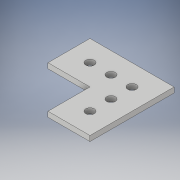
# Autodesk Inventor part: 8020 connector
Saved by Autodesk Inventor 2018 (Build 220112000, 112)
## iProperties
Created: 2019-01-26
Part Number: 8020 connector
Material: Generic
Document SubType Name: Modeling
Designer: s-2513225
Density: 1 g/cm^3
Appearance: Default
Author: s-2513225
Autodesk Inventor part; units mm, degrees
ref_plane "YZ Plane" through (0, 0, 0) normal (1, 0, 0) x (0, 1, 0)
ref_plane "XZ Plane" through (0, 0, 0) normal (0, 1, 0) x (-1, 0, 0)
ref_plane "XY Plane" through (0, 0, 0) normal (0, 0, 1) x (1, 0, 0)
sketch "Sketch1" plane through (0, 0, 0) normal (0, 1, 0) x (-1, 0, 0)
  line L0 (0, 0) -> (25.4, 0)
  line L1 (25.4, 0) -> (25.4, -25.4)
  line L2 (25.4, -50.8) -> (0, -50.8)
  line L3 (0, -50.8) -> (0, 0)
  line L4 (25.4, -50.8) -> (50.8, -50.8)
  line L5 (50.8, -50.8) -> (50.8, -25.4)
  line L6 (50.8, -25.4) -> (25.4, -25.4)
  line L7 (12.7, 0) -> (12.7, -12.7) construction
  line L8 (12.7, -12.7) -> (12.7, -25.4) construction
  line L9 (12.7, -25.4) -> (12.7, -38.1) construction
  line L10 (12.7, -38.1) -> (25.4, -38.1) construction
  line L11 (25.4, -38.1) -> (38.1, -38.1) construction
  line L12 (38.1, -38.1) -> (50.8, -38.1) construction
  circle A0 centre (12.7, -12.7) radius 2.5797
  circle A1 centre (12.7, -25.4) radius 2.5797
  circle A2 centre (12.7, -38.1) radius 2.5797
  circle A3 centre (25.4, -38.1) radius 2.5797
  circle A4 centre (38.1, -38.1) radius 2.5797
  dimension "d0" = 25.4
  dimension "d2" = 25.4
  dimension "d3" = 25.4
  dimension "d4" = 12.7
  dimension "d5" = 12.7
  dimension "d6" = 12.7
  dimension "d7" = 5.1594
  dimension "d8" = 5.1594
  dimension "d9" = 5.1594
  dimension "d10" = 5.1594
  dimension "d11" = 5.1594
  constraints: 26 end point, 5 centre point, 5 coincident, 3 parallel, 3 point on line, 2 horizontal, 2 midpoint, 2 perpendicular, 1 vertical
  measures "d0" distance of L2.start L2.end
  measures "d2" distance of L1.end L5.end
  measures "d3" distance of L5.end L4.end
  measures "d4" distance of L7.start L7.end
  measures "d5" distance of L7.end L8.end
  measures "d6" distance of L8.end L9.end
  measures "d7" diameter of A0
  measures "d8" diameter of A1
  measures "d9" diameter of A2
  measures "d10" diameter of A3
  measures "d11" diameter of A4
extrude "Extrusion1" add sketch "Sketch1" along normal blind 3.175
body "Solid1"
